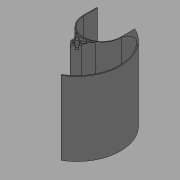
# Autodesk Inventor part: inner_mechanism
Saved by Autodesk Inventor 2019 (Build 230136000, 136)
## iProperties
Part Number: inner_mechanism
Material: Generic
Document SubType Name: Modeling
Designer: Javi
Appearance: Default
Mass: 408.244 g
Surface Area: 2031.36 cm^2
Volume: 408.244 cm^3
Density: 1 g/cm^3
Author: Javi
Autodesk Inventor part; units mm, degrees
ref_plane "YZ Plane" through (0, 0, 0) normal (1, 0, 0) x (0, 1, 0)
ref_plane "XZ Plane" through (0, 0, 0) normal (0, 1, 0) x (-1, 0, 0)
ref_plane "XY Plane" through (0, 0, 0) normal (0, 0, 1) x (1, 0, 0)
sketch "Sketch1" plane through (0, 0, 0) normal (0, 1, 0) x (-1, 0, 0)
  circle A0 centre (0, 0) radius 120
  dimension "d0" = 240
  constraints: 1 centre point, 1 coincident
  measures "d0" diameter of A0
extrude "Extrusion1" add sketch "Sketch1" along normal blind 200
sketch "Sketch2" plane through (0, 200, 0) normal (0, 1, 0) x (1, 0, 0)
  arc A0 (0, 18) -> (50, 68) centre (0, 68) ccw
  circle A1 centre (0, 0) radius 120 projected
  circle A2 centre (0, 0) radius 120
  line L0 (120, 0) -> (125, 0) construction
  line L1 (52, 68) -> (50, 68)
  arc A3 (-13, 0) -> (13, 0) centre (0, 0) ccw
  arc A4 (26.2581, 23.1167) -> (52, 68) centre (0, 68) ccw
  line L2 (50, 68) -> (50, 106.8831)
  line L3 (50, 68) -> (88.8831, 68) construction
  arc A5 (-50, 68) -> (50, 68) centre (0, 68) ccw
  line L4 (-13, 0) -> (13, 0)
  line L5 (-52, 68) -> (-52, 105.9245)
  line L6 (-50, 68) -> (-50, 105.9245)
  line L7 (-50, 105.9245) -> (-52, 105.9245)
  arc A6 (59, -102.191) -> (50, 106.8831) centre (0, 0) ccw
  arc A7 (57.5, -99.5929) -> (82.2894, 80.3334) centre (0, 0) ccw
  arc A8 (82.2894, 80.3334) -> (52, 68) centre (69.6557, 68) ccw
  line L8 (57.5, -99.5929) -> (59, -102.191)
  arc A9 (-13, 0) -> (-26.2581, 23.1167) centre (-39.7821, 0) ccw
  arc A10 (26.2581, 23.1167) -> (13, 0) centre (39.7821, 0) ccw
  arc A11 (-52, 68) -> (-26.2581, 23.1167) centre (0, 68) ccw
  arc A12 (26.2581, 23.1167) -> (52, 68) centre (0, 68) ccw
  dimension "d21" = 13
  dimension "d23" = 2
  dimension "d32" = 90
  dimension "d33" = 50
  dimension "d57" = 68
  dimension "d58" = 236
  dimension "d59" = 0
  dimension "d60" = 230
  dimension "d61" = 30
  dimension "d62" = 0
  dimension "d63" = 2
  dimension "d64" = 37.9245
  constraints: 22 point on circle, 18 end point, 11 centre point, 8 tangent, 7 coincident, 5 horizontal, 2 line through centre, 1 concentric, 1 horizontal alignment, 1 parallel, 1 perpendicular, 1 point on line, 1 vertical, 3 other
  measures "d21" radius of A3
  measures "d23" distance of L1.end L1.start
  measures "d32" angle of L3 L2
  measures "d33" radius of A0
  measures "d57" distance of A0.centre point (0, 0)
  measures "d58" diameter of A6
  measures "d59" horizontal distance of point (0, 0) A0.centre
  measures "d60" diameter of A7
  measures "d61" angle of L2 L8
  measures "d62" distance from line of point (0, 0) L4
  measures "d63" distance between parallel lines of L6 L5
  measures "d64" distance of L5.start L5.end
extrude "Extrusion3" cut sketch "Sketch2" against normal through all
sketch "Sketch3" plane through (0, 0, 0) normal (0, -1, 0) x (1, 0, 0)
  circle A0 centre (0, 0) radius 11.5
  dimension "d42" = 23
  constraints: 1 centre point, 1 coincident
  measures "d42" diameter of A0
extrude "Extrusion4" cut sketch "Sketch3" against normal blind 17
sketch "Sketch5" plane through (0, 17, 0) normal (0, -1, 0) x (1, 0, 0)
  circle A0 centre (0, 0) radius 7.5
  dimension "d46" = 15
  constraints: 1 centre point, 1 coincident
  measures "d46" diameter of A0
extrude "Extrusion5" cut sketch "Sketch5" against normal blind 8
sketch "Sketch6" plane through (0, 25, 0) normal (0, -1, 0) x (1, 0, 0)
  circle A0 centre (0, 0) radius 4.5
  dimension "d49" = 9
  constraints: 1 centre point, 1 coincident
  measures "d49" diameter of A0
extrude "Extrusion6" cut sketch "Sketch6" against normal blind 165
derived "Parallax-Servo-Horn.ipt"
sketch "Sketch1_1" plane through (0, 17.3761, 0) normal (0, 0, 1) x (1, 0, 0)
  line L0 (17.8043, -15.3923) -> (7.873, -13.2486)
  line L1 (7.873, -13.2486) -> (6.3161, -13.2486)
  arc A0 (4.1275, -11.06) -> (6.3161, -13.2486) centre (6.3161, -11.06) ccw
  line L2 (4.1275, -11.06) -> (4.1275, -9.5031)
  line L3 (4.1275, -9.5031) -> (1.9838, 0.4282)
  arc A1 (1.9838, 0.4282) -> (-1.9838, 0.4282) centre (0, 0) ccw
  line L4 (-1.9838, 0.4282) -> (-4.1275, -9.5031)
  line L5 (-4.1275, -9.5031) -> (-4.1275, -11.06)
  arc A2 (-6.3161, -13.2486) -> (-4.1275, -11.06) centre (-6.3161, -11.06) ccw
  line L6 (-6.3161, -13.2486) -> (-7.873, -13.2486)
  line L7 (-7.873, -13.2486) -> (-17.8043, -15.3923)
  arc A3 (-17.8043, -15.3923) -> (-17.8043, -19.3599) centre (-17.3761, -17.3761) ccw
  line L8 (-17.8043, -19.3599) -> (-7.873, -21.5036)
  line L9 (-7.873, -21.5036) -> (-6.3161, -21.5036)
  arc A4 (-4.1275, -23.6922) -> (-6.3161, -21.5036) centre (-6.3161, -23.6922) ccw
  line L10 (-4.1275, -23.6922) -> (-4.1275, -25.2491)
  line L11 (-4.1275, -25.2491) -> (-1.9838, -35.1804)
  arc A5 (-1.9838, -35.1804) -> (1.9838, -35.1804) centre (0, -34.7522) ccw
  line L12 (1.9838, -35.1804) -> (4.1275, -25.2491)
  line L13 (4.1275, -25.2491) -> (4.1275, -23.6922)
  arc A6 (6.3161, -21.5036) -> (4.1275, -23.6922) centre (6.3161, -23.6922) ccw
  line L14 (6.3161, -21.5036) -> (7.873, -21.5036)
  line L15 (7.873, -21.5036) -> (17.8043, -19.3599)
  arc A7 (17.8043, -19.3599) -> (17.8043, -15.3923) centre (17.3761, -17.3761) ccw
  circle A8 centre (0, -9.2735) radius 0.635
  circle A9 centre (-0.0143, -6.3525) radius 0.635
  circle A10 centre (-0.0286, -3.4316) radius 0.635
  circle A11 centre (-0.0428, -0.5106) radius 0.635
  circle A12 centre (-16.8655, -17.4189) radius 0.635
  circle A13 centre (-13.9445, -17.4047) radius 0.635
  circle A14 centre (-11.0236, -17.3904) radius 0.635
  circle A15 centre (-8.1026, -17.3761) radius 0.635
  circle A16 centre (0.0428, -34.2416) radius 0.635
  circle A17 centre (0.0286, -31.3206) radius 0.635
  circle A18 centre (0.0143, -28.3997) radius 0.635
  circle A19 centre (0, -25.4787) radius 0.635
  circle A20 centre (16.8655, -17.3333) radius 0.635
  circle A21 centre (13.9445, -17.3475) radius 0.635
  circle A22 centre (11.0236, -17.3618) radius 0.635
  circle A23 centre (8.1026, -17.3761) radius 0.635
  circle A24 centre (0, -17.3761) radius 4.7016
sketch "Sketch11" plane through (0, 200, 0) normal (0, 1, 0) x (1, 0, 0)
  arc A0 (-13, 0) -> (13, 0) centre (0, 0) ccw projected
  arc A1 (26.2581, 23.1167) -> (13, 0) centre (39.7821, 0) ccw projected
  arc A2 (26.2581, 23.1167) -> (52, 68) centre (0, 68) ccw projected
  arc A3 (82.2894, 80.3334) -> (52, 68) centre (69.6557, 68) ccw projected
  arc A4 (57.5, -99.5929) -> (82.2894, 80.3334) centre (0, 0) ccw projected
  line L0 (57.5, -99.5929) -> (59, -102.191) projected
  arc A5 (59, -102.191) -> (50, 106.8831) centre (0, 0) ccw projected
  line L1 (50, 106.8831) -> (50, 68) projected
  arc A6 (-50, 68) -> (50, 68) centre (0, 68) ccw projected
  line L2 (-50, 68) -> (-50, 105.9245) projected
  line L3 (-50, 105.9245) -> (-52, 105.9245) projected
  line L4 (-52, 105.9245) -> (-52, 68) projected
  arc A7 (-52, 68) -> (-26.2581, 23.1167) centre (0, 68) ccw projected
  arc A8 (-13, 0) -> (-26.2581, 23.1167) centre (-39.7821, 0) ccw projected
  arc A9 (-13, 0) -> (-26.2581, 23.1167) centre (-39.7821, 0) ccw projected
  arc A10 (26.2581, 23.1167) -> (13, 0) centre (39.7821, 0) ccw projected
  arc A11 (-26.2581, 23.1167) -> (26.2581, 23.1167) centre (0, 68) ccw
  dimension "d71" = 52
  constraints: 2 point on circle, 1 centre point
  measures "d71" radius of A11
extrude "Extrusion8" cut sketch "Sketch11" against normal blind 3 contours A8 A11 A1 A0
sketch "Sketch12" plane through (0, 197, 0) normal (0, 1, 0) x (1, 0, 0)
  line L0 (11.1868, 13.9923) -> (2.6485, 8.4857)
  line L1 (2.6485, 8.4857) -> (1.5475, 7.3847)
  arc A0 (-1.5475, 7.3847) -> (1.5475, 7.3847) centre (0, 8.9323) ccw
  line L2 (-1.5475, 7.3847) -> (-2.6485, 8.4857)
  line L3 (-2.6485, 8.4857) -> (-11.1868, 13.9923)
  arc A1 (-11.1868, 13.9923) -> (-13.9923, 11.1868) centre (-12.2868, 12.2868) ccw
  line L4 (-13.9923, 11.1868) -> (-8.4857, 2.6485)
  line L5 (-8.4857, 2.6485) -> (-7.3847, 1.5475)
  arc A2 (-7.3847, -1.5475) -> (-7.3847, 1.5475) centre (-8.9323, 0) ccw
  line L6 (-7.3847, -1.5475) -> (-8.4857, -2.6485)
  line L7 (-8.4857, -2.6485) -> (-13.9923, -11.1868)
  arc A3 (-13.9923, -11.1868) -> (-11.1868, -13.9923) centre (-12.2868, -12.2868) ccw
  line L8 (-11.1868, -13.9923) -> (-2.6485, -8.4857)
  line L9 (-2.6485, -8.4857) -> (-1.5475, -7.3847)
  arc A4 (1.5475, -7.3847) -> (-1.5475, -7.3847) centre (0, -8.9323) ccw
  line L10 (1.5475, -7.3847) -> (2.6485, -8.4857)
  line L11 (2.6485, -8.4857) -> (11.1868, -13.9923)
  arc A5 (11.1868, -13.9923) -> (13.9923, -11.1868) centre (12.2868, -12.2868) ccw
  line L12 (13.9923, -11.1868) -> (8.4857, -2.6485)
  line L13 (8.4857, -2.6485) -> (7.3847, -1.5475)
  arc A6 (7.3847, 1.5475) -> (7.3847, -1.5475) centre (8.9323, 0) ccw
  line L14 (7.3847, 1.5475) -> (8.4857, 2.6485)
  line L15 (8.4857, 2.6485) -> (13.9923, 11.1868)
  arc A7 (13.9923, 11.1868) -> (11.1868, 13.9923) centre (12.2868, 12.2868) ccw
  line L16 (2.3327, 8.8769) -> (10.9158, 14.4125)
  arc A8 (14.4125, 10.9158) -> (10.9158, 14.4125) centre (12.2868, 12.2868) ccw
  line L17 (14.4125, 10.9158) -> (8.8769, 2.3327)
  line L18 (8.8769, 2.3327) -> (7.7383, 1.194)
  arc A9 (7.7383, 1.194) -> (7.7383, -1.194) centre (8.9323, 0) ccw
  line L19 (7.7383, -1.194) -> (8.8769, -2.3327)
  line L20 (8.8769, -2.3327) -> (14.4125, -10.9158)
  arc A10 (10.9158, -14.4125) -> (14.4125, -10.9158) centre (12.2868, -12.2868) ccw
  line L21 (10.9158, -14.4125) -> (2.3327, -8.8769)
  line L22 (2.3327, -8.8769) -> (1.194, -7.7383)
  arc A11 (1.194, -7.7383) -> (-1.194, -7.7383) centre (0, -8.9323) ccw
  line L23 (-1.194, -7.7383) -> (-2.3327, -8.8769)
  line L24 (-2.3327, -8.8769) -> (-10.9158, -14.4125)
  arc A12 (-14.4125, -10.9158) -> (-10.9158, -14.4125) centre (-12.2868, -12.2868) ccw
  line L25 (-14.4125, -10.9158) -> (-8.8769, -2.3327)
  line L26 (-8.8769, -2.3327) -> (-7.7383, -1.194)
  arc A13 (-7.7383, -1.194) -> (-7.7383, 1.194) centre (-8.9323, 0) ccw
  line L27 (-7.7383, 1.194) -> (-8.8769, 2.3327)
  line L28 (-8.8769, 2.3327) -> (-14.4125, 10.9158)
  arc A14 (-10.9158, 14.4125) -> (-14.4125, 10.9158) centre (-12.2868, 12.2868) ccw
  line L29 (-10.9158, 14.4125) -> (-2.3327, 8.8769)
  line L30 (-2.3327, 8.8769) -> (-1.194, 7.7383)
  arc A15 (-1.194, 7.7383) -> (1.194, 7.7383) centre (0, 8.9323) ccw
  line L31 (1.194, 7.7383) -> (2.3327, 8.8769)
  point P0 (0, 0)
  point P1 (0, 0)
  dimension "d32" = 90
  dimension "d74" = 0.5
  constraints: 64 end point, 32 point on circle, 16 centre point, 23 other
  measures "d74" distance between parallel lines of L0 L16
extrude "Extrusion9" cut sketch "Sketch12" against normal blind 9 contours A7 L15 L14 A6 L13 L12 A5 L11 L10 A4 L9 L8 A3 L7 L6 A2 L5 L4 A1 L3 L2 A0 L1 L0 | L16 A8 L17 L18 A9 L19 L20 A10 L21 L22 A11 L23 L24 A12 L25 L26 A13 L27 L28 A14 L29 L30 A15 L31
body "Solid1"
